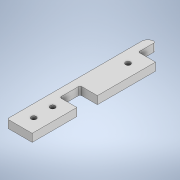
# Autodesk Inventor part: Lower slide
Saved by Autodesk Inventor 2021 (Build 250183000, 183)
## iProperties
Created: 2020-08-14
Part Number: Lower slide
Material: Generic
Document SubType Name: Modeling
Designer: jgray
Density: 1 g/cm^3
Appearance: Default
Author: jgray
Autodesk Inventor part; units mm, degrees
ref_plane "YZ Plane" through (0, 0, 0) normal (1, 0, 0) x (0, 1, 0)
ref_plane "XZ Plane" through (0, 0, 0) normal (0, 1, 0) x (-1, 0, 0)
ref_plane "XY Plane" through (0, 0, 0) normal (0, 0, 1) x (1, 0, 0)
sketch "Sketch1" plane through (0, 0, 0) normal (0, 1, 0) x (-1, 0, 0)
  line L0 (0, 0) -> (15.9, 0)
  line L1 (15.9, -16) -> (15.9, -100.5)
  line L2 (10, -104.5) -> (0, -104.5)
  line L3 (0, -104.5) -> (0, 0)
  line L4 (0, -104.5) -> (11, -104.5)
  line L5 (11, -103.5) -> (11, -94.5)
  line L6 (10, -93.5) -> (0, -93.5)
  line L7 (0, -93.5) -> (0, -104.5)
  line L8 (10, -43.5) -> (0, -43.5)
  line L9 (0, -43.5) -> (0, -56.5)
  line L10 (0, -56.5) -> (10, -56.5)
  line L11 (11, -55.5) -> (11, -44.5)
  line L12 (15.9, 0) -> (0, 0)
  line L13 (0, 0) -> (0, -15)
  line L14 (0, -15) -> (14.9, -15)
  line L15 (15.9, -15) -> (15.9, 0)
  arc A0 (11.9, -104.5) -> (15.9, -100.5) centre (11.9, -100.5) ccw
  arc A1 (15.9, -16) -> (14.9, -15) centre (14.9, -16) ccw
  arc A2 (11, -44.5) -> (10, -43.5) centre (10, -44.5) ccw
  arc A3 (10, -56.5) -> (11, -55.5) centre (10, -55.5) ccw
  arc A4 (11, -94.5) -> (10, -93.5) centre (10, -94.5) ccw
  line L16 (11.9, -104.5) -> (12, -104.5)
  arc A5 (11, -103.5) -> (12, -104.5) centre (12, -103.5) ccw
  point P0 (15.9, -104.5)
  point P1 (11, -93.5)
  point P2 (11, -43.5)
  point P3 (11, -56.5)
  point P4 (0, -43.5)
  point P5 (0, -56.5)
  point P6 (11.9667, -104.4994)
  dimension "d0" = 15.9
  dimension "d1" = 104.5
  dimension "d2" = 11
  dimension "d3" = 11
  dimension "d4" = 11
  dimension "d5" = 13
  dimension "d6" = 56.5
  dimension "d7" = 15
  dimension "d8" = 4
  dimension "d9" = 1
  dimension "d22" = 1
  constraints: 34 end point, 16 point on line, 12 point on circle, 12 tangent, 8 parallel, 6 centre point, 5 horizontal, 4 perpendicular, 3 equal radius
  measures "d0" distance of point (15.9, -104.5) L2.end
  measures "d1" distance of L0.end point (15.9, -104.5)
  measures "d2" distance of L6.end point (11, -93.5)
  measures "d3" distance of point (11, -93.5) L4.end
  measures "d4" distance of point (11, -56.5) L9.end
  measures "d5" distance of L9.end L8.end
  measures "d6" distance between parallel lines of L0 L10
  measures "d7" distance of L13.end L12.end
  measures "d8" radius of A0
  measures "d9" radius of A1
  measures "d22" radius of A5
extrude "Extrusion1" add sketch "Sketch1" along normal blind 5 contours L1 A0 A5 L5 A4 L6 L3 L10 A3 L11 A2 L8 L14 A1
sketch "Sketch2" plane through (0, 5, 0) normal (0, 1, 0) x (1, 0, 0)
  line L0 (-8, -6.918) -> (-8, 116.4057) construction
  line L1 (0, 15) -> (0, 43.5) construction
  point P0 (0, 0)
  point P1 (-8, 84)
  point P2 (-8, 36)
  point P3 (-8, 24)
  dimension "d12" = 8
  dimension "d13" = 36
  dimension "d14" = 84
  dimension "d23" = 24
  constraints: 3 point on line, 2 end point, 1 vertical
  measures "d12" distance between parallel lines of L1 L0
  measures "d13" vertical distance of point (-8, 36) point (0, 0)
  measures "d14" vertical distance of point (0, 0) point (-8, 84)
  measures "d23" vertical distance of point (0, 0) point (-8, 24)
hole "Hole1" at (-8, 5, -84) at (-8, 5, -36) at (-8, 5, -24) direction (0, -1, 0) diameter 3.2 end through all
body "Solid1"
